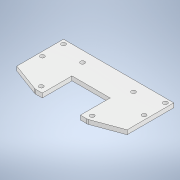
# Autodesk Inventor part: Chassis
Saved by Autodesk Inventor 2022.3 (Build 263350000, 350)
## iProperties
Created: 2022-05-26
Part Number: Chassis
Material: UHMW, White
Document SubType Name: Modeling
Designer: Nathan Cai
Density: 0.94 g/cm^3
Appearance: Smooth - White
Mass: 325.409 g
Surface Area: 397.42 cm^2
Volume: 271.174 cm^3
Author: Nathan Cai
Autodesk Inventor part; units mm, degrees
ref_plane "YZ Plane" through (0, 0, 0) normal (1, 0, 0) x (0, 1, 0)
ref_plane "XZ Plane" through (0, 0, 0) normal (0, 1, 0) x (-1, 0, 0)
ref_plane "XY Plane" through (0, 0, 0) normal (0, 0, 1) x (1, 0, 0)
sketch "Sketch1" plane through (0, 0, 0) normal (0, 1, 0) x (-1, 0, 0)
  line L0 (82.55, 34.925) -> (-82.55, 34.925) construction
  line L1 (-82.55, 34.925) -> (-82.55, -34.925)
  line L2 (-82.55, -34.925) -> (82.55, -34.925)
  line L3 (82.55, -34.925) -> (82.55, 34.925)
  line L4 (82.55, 34.925) -> (-82.55, -34.925) construction
  line L5 (-82.55, 34.925) -> (82.55, -34.925) construction
  line L6 (-28.575, 63.5) -> (28.575, 63.5) construction
  line L7 (28.575, 63.5) -> (28.575, 6.35)
  line L8 (28.575, 6.35) -> (-28.575, 6.35)
  line L9 (-28.575, 6.35) -> (-28.575, 63.5)
  line L10 (-28.575, 63.5) -> (28.575, 6.35) construction
  line L11 (28.575, 63.5) -> (-28.575, 6.35) construction
  circle A0 centre (-38.1, 42.8625) radius 3.175
  line L12 (0, 34.925) -> (0, -34.925) construction
  circle A1 centre (-38.1, 42.8625) radius 7.9375
  line L13 (-38.1, 50.8) -> (-28.575, 50.8)
  circle A2 centre (38.1, 42.8625) radius 3.175
  circle A3 centre (38.1, 42.8625) radius 7.9375
  line L14 (38.1, 50.8) -> (28.575, 50.8)
  circle A4 centre (-76.2, -28.575) radius 3.175
  circle A5 centre (-76.2, 3.175) radius 3.175
  circle A6 centre (76.2, -28.575) radius 3.175
  circle A7 centre (76.2, 3.175) radius 3.175
  line L15 (-82.55, 34.925) -> (-40.8472, 50.3094)
  line L16 (82.55, 34.925) -> (40.8472, 50.3094)
  circle A8 centre (-38.1, -19.05) radius 3.175
  circle A9 centre (38.1, -19.05) radius 3.175
  circle A10 centre (-38.1, -19.05) radius 6.35
  circle A11 centre (38.1, -19.05) radius 6.35
  point P0 (0, 0)
  point P1 (28.575, 34.925)
  point P2 (-28.575, 34.925)
  point P3 (-50.8, 34.925)
  point P4 (28.575, 50.8)
  point P5 (40.8472, 50.3094)
  dimension "d0" = 165.1
  dimension "d1" = 69.85
  dimension "d4" = 57.15
  dimension "d6" = 6.35
  dimension "d7" = 38.1
  dimension "d8" = 15.875
  dimension "d9" = 31.75
  dimension "d10" = 6.35
  dimension "d11" = 6.35
  dimension "d12" = 6.35
  dimension "d13" = 31.75
  dimension "d14" = 6.35
  dimension "d15" = 6.35
  dimension "d16" = 6.35
  dimension "d17" = 9.525
  dimension "d18" = 15.875
  dimension "d19" = 12.7
  dimension "d20" = 44.45
  constraints: 34 end point, 11 centre point, 9 symmetric about line, 6 midpoint, 4 parallel, 3 coincident, 3 perpendicular, 3 tangent, 2 horizontal, 2 point on circle, 2 point on line, 9 other
  measures "d0" distance of L2.end L1.end
  measures "d1" distance between parallel lines of L0 L2
  measures "d4" distance of L7.end L8.end
  measures "d6" diameter of A0
  measures "d7" distance from line of L12 A0.centre
  measures "d8" diameter of A1
  measures "d9" distance from line of L1 point (-50.8, 34.925)
  measures "d10" diameter of A4
  measures "d11" diameter of A5
  measures "d12" distance from line of L2 A4.centre
  measures "d13" distance of A4.centre A5.centre
  measures "d14" distance from line of L1 A4.centre
  measures "d15" distance from line of L1 A5.centre
  measures "d16" diameter of A8
  measures "d17" distance from line of L9 A8.centre
  measures "d18" distance from line of L2 A8.centre
  measures "d19" diameter of A10
  measures "d20" distance between parallel lines of L8 L14
extrude "Extrusion1" add sketch "Sketch1" along normal blind 6.35 contours L15 A1 L13 L9 L8 L7 L14 A3 L16 L3 L2 L1 | A1 | A3 | A10 | A11
equation "\"d15\" = d14"
body "Solid1"
